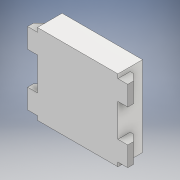
# Autodesk Inventor part: Nes_Led
Saved by Autodesk Inventor 2017 (Build 210142000, 142)
## iProperties
Created: 2018-11-04
Part Number: Nes_Led
Material: Generic
Document SubType Name: Modeling
Designer: ludov
Density: 1 g/cm^3
Appearance: Default
Author: ludov
Autodesk Inventor part; units mm, degrees
ref_plane "YZ Plane" through (0, 0, 0) normal (1, 0, 0) x (0, 1, 0)
ref_plane "XZ Plane" through (0, 0, 0) normal (0, 1, 0) x (-1, 0, 0)
ref_plane "XY Plane" through (0, 0, 0) normal (0, 0, 1) x (1, 0, 0)
sketch "Esquisse1" plane through (0, 0, 0) normal (0, 1, 0) x (-1, 0, 0)
  line L0 (0, 0) -> (-4.9, 0)
  line L1 (-4.9, 0) -> (-4.9, -4.9)
  line L2 (-4.9, -4.9) -> (0, -4.9)
  line L3 (0, -4.9) -> (0, 0)
  dimension "d0" = 4.9
  constraints: 8 end point, 2 parallel, 2 perpendicular, 1 horizontal
  measures "d0" distance between parallel lines of L3 L1
extrude "Extrusion1" add sketch "Esquisse1" along normal blind 1.4
sketch "Esquisse2" plane through (0, 0, -4.9) normal (-1, 0, 0) x (0, 0, 1)
  line L0 (0.25, 0.75) -> (1.45, 0.75)
  line L1 (1.45, 0.75) -> (1.45, 0)
  line L2 (1.45, 0) -> (0.25, 0)
  line L3 (0.25, 0) -> (0.25, 0.75)
  line L4 (0, 0) -> (0, 1.4) projected
  line L5 (0, 0) -> (4.9, 0) projected
  dimension "d4" = 1.2
  dimension "d5" = 0.75
  dimension "d8" = 0.25
  dimension "d9" = 0
  constraints: 8 end point, 2 parallel, 1 horizontal, 1 perpendicular
  measures "d4" distance between parallel lines of L1 L3
  measures "d5" distance between parallel lines of L0 L2
  measures "d8" distance from line of L4 L2.end
  measures "d9" distance from line of L5 L2.end
extrude "Extrusion2" add sketch "Esquisse2" along normal blind 0.6
chamfer "Chanfrein1" distance 0.4 angle 45 1 edges at (-0.6, 0.75, -4.05)
sketch "Esquisse3" plane through (0, 0, 0) normal (-1, 0, 0) x (0, 0, 1)
  line L0 (-1.45, 0.75) -> (-0.25, 0.75)
  line L1 (-0.25, 0.75) -> (-0.25, 0)
  line L2 (-0.25, 0) -> (-1.45, 0)
  line L3 (-1.45, 0) -> (-1.45, 0.75)
  line L4 (-3.45, 0) -> (0, 0) projected
  line L5 (0, 0) -> (0, 1.4) projected
  dimension "d15" = 0
  dimension "d16" = 0.75
  dimension "d17" = 1.2
  dimension "d18" = 0.25
  constraints: 8 end point, 2 parallel, 1 horizontal, 1 perpendicular
  measures "d15" distance from line of L4 L1.end
  measures "d16" distance of L2.end L0.start
  measures "d17" distance of L0.start L0.end
  measures "d18" distance from line of L5 L1.end
extrude "Extrusion3" add sketch "Esquisse3" along normal blind 0.6
chamfer "Chanfrein2" distance 0.4 angle 45 1 edges at (-0.6, 0.75, -0.85)
sketch "Esquisse4" plane through (4.9, 0, 0) normal (1, 0, 0) x (0, 0, -1)
  line L0 (0.25, 0.75) -> (1.45, 0.75)
  line L1 (1.45, 0.75) -> (1.45, 0)
  line L2 (1.45, 0) -> (0.25, 0)
  line L3 (0.25, 0) -> (0.25, 0.75)
  point P0 (0, 0)
  dimension "d24" = 0.75
  dimension "d25" = 1.2
  dimension "d26" = 0
  dimension "d27" = 0.25
  constraints: 8 end point, 2 parallel, 1 horizontal, 1 perpendicular
  measures "d24" distance of L2.end L0.start
  measures "d25" distance of L0.start L0.end
  measures "d26" distance from line of L2 point (0, 0)
  measures "d27" distance from line of L3 point (0, 0)
extrude "Extrusion4" add sketch "Esquisse4" along normal blind 0.6
chamfer "Chanfrein3" distance 0.4 angle 45 1 edges at (5.5, 0.75, -0.85)
sketch "Esquisse5" plane through (4.9, 0, -4.9) normal (1, 0, 0) x (0, 0, -1)
  line L0 (-1.45, 0.75) -> (-0.25, 0.75)
  line L1 (-0.25, 0.75) -> (-0.25, 0)
  line L2 (-0.25, 0) -> (-1.45, 0)
  line L3 (-1.45, 0) -> (-1.45, 0.75)
  line L4 (-3.45, 0) -> (0, 0) projected
  line L5 (0, 0) -> (0, 1.4) projected
  point P0 (-4.9, 0)
  dimension "d33" = 1.2
  dimension "d34" = 0.75
  dimension "d35" = 0
  dimension "d36" = 0.25
  constraints: 8 end point, 2 parallel, 1 horizontal, 1 perpendicular
  measures "d33" distance of L0.start L0.end
  measures "d34" distance of L2.end L0.start
  measures "d35" distance from line of L4 L1.end
  measures "d36" distance from line of L5 L1.end
extrude "Extrusion5" add sketch "Esquisse5" along normal blind 0.6
chamfer "Chanfrein4" distance 0.4 angle 45 1 edges at (5.5, 0.75, -4.05)
sketch "Esquisse8" plane through (0, 1.4, 0) normal (0, 1, 0) x (1, 0, 0)
  line L0 (4.9, 4.9) -> (0, 4.9) projected
  line L1 (0.8, 4.9) -> (4.9, 4.9)
  line L2 (4.9, 4.9) -> (4.9, 0)
  line L3 (4.9, 0) -> (0, 0)
  line L4 (0, 0) -> (0, 4.1)
  line L5 (0, 4.65) -> (0, 3.45) projected
  line L6 (0.8, 4.9) -> (0, 4.1)
  dimension "d44" = 0.8
  dimension "d45" = 0.8
  constraints: 10 end point, 2 perpendicular, 2 point on line, 1 horizontal
  measures "d44" distance of L0.end L1.start
  measures "d45" distance of L0.end L4.end
extrude "Extrusion6" add sketch "Esquisse8" along normal blind 0.1
